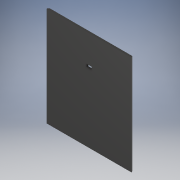
# Autodesk Inventor part: BA03
Saved by Autodesk Inventor 2017 (Build 210142000, 142)
## iProperties
Created: 2018-10-18
Part Number: BA03
Material: ABS Plastic
Document SubType Name: Modeling
Designer: Dell
Density: 1.06 g/cm^3
Appearance: Smooth - Black
Author: Dell
Autodesk Inventor part; units mm, degrees
ref_plane "YZ Plane" through (0, 0, 0) normal (1, 0, 0) x (0, 1, 0)
ref_plane "XZ Plane" through (0, 0, 0) normal (0, 1, 0) x (-1, 0, 0)
ref_plane "XY Plane" through (0, 0, 0) normal (0, 0, 1) x (1, 0, 0)
sketch "Sketch1" plane through (0, 0, 0) normal (0, 0, 1) x (1, 0, 0)
  line L0 (0, 0) -> (296.3316, 0)
  line L1 (296.3316, 0) -> (296.3316, -355.6)
  line L2 (296.3316, -355.6) -> (0, -355.6)
  line L3 (0, -355.6) -> (0, 0)
  dimension "d0" = 296.3316
  dimension "d1" = 355.6
  constraints: 8 end point, 2 parallel, 1 horizontal, 1 perpendicular
  measures "d0" distance of L1.end L2.end
  measures "d1" distance of L0.end L1.end
extrude "Extrusion1" add sketch "Sketch1" along normal blind 6.35
sketch "Sketch2" plane through (0, 0, 0) normal (0, 1, 0) x (1, 0, 0)
  line L0 (296.3316, -6.35) -> (0, -6.35) projected
  line L1 (0, -6.35) -> (-3.6662, -6.35)
  line L2 (-3.6662, -6.35) -> (0, 0)
  line L3 (0, 0) -> (0, -6.35) projected
  line L4 (0, 0) -> (0, -6.35) projected
  line L5 (0, -6.35) -> (0, 0)
  line L6 (296.3316, -6.35) -> (299.9978, -6.35)
  line L7 (296.3316, 0) -> (296.3316, -6.35) projected
  line L8 (299.9978, -6.35) -> (296.3316, 0)
  line L9 (296.3316, 0) -> (296.3316, -6.35)
  dimension "d4" = 30
  dimension "d5" = 60
  constraints: 12 end point, 2 collinear, 2 horizontal
  measures "d4" angle of L3 L2
  measures "d5" angle of L6 L8
extrude "Extrusion2" add sketch "Sketch2" against normal blind 355.6
sketch "Sketch5" plane through (0, 0, 6.35) normal (0, 0, 1) x (1, 0, 0)
  line L0 (139.1658, -100) -> (157.1658, -100)
  line L1 (157.1658, -100) -> (157.1658, -110)
  line L2 (157.1658, -110) -> (139.1658, -110)
  line L3 (139.1658, -110) -> (139.1658, -100)
  line L4 (-3.6662, 0) -> (299.9978, 0) projected
  point P0 (0, 0)
  point P1 (148.1658, -100)
  point P2 (148.1658, 0)
  dimension "d77" = 18
  dimension "d78" = 10
  dimension "d79" = 100
  constraints: 8 end point, 2 midpoint, 2 parallel, 1 horizontal, 1 perpendicular, 1 vertical alignment
  measures "d77" distance of L1.end L2.end
  measures "d78" distance of L0.end L1.end
  measures "d79" distance between parallel lines of L4 L0
extrude "Extrusion5" cut sketch "Sketch5" against normal through all
body "Solid1"
